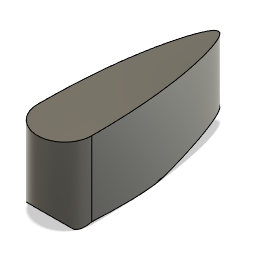
DLG_Höhenruder_träger (Autodesk Fusion 360 design; units mm, degrees)
Autodesk Fusion 360 part; units mm, degrees
sketch "Skizze1" plane through (0, 0, 0) normal (0, 0, 1) x (1, 0, 0)
  line L0 (6, 10) -> (-6, 10)
  line L1 (-6, 10) -> (-6, -10)
  line L2 (-6, -10) -> (6, -10)
  line L3 (6, -10) -> (6, 10)
  line L4 (6, 10) -> (-6, -10) construction
  line L5 (-6, 10) -> (6, -10) construction
  dimension "d1" = 12
  dimension "d2" = 20
  constraint horizontal L0
  constraint perpendicular L0 L1
  constraint parallel L0 L2
  constraint parallel L1 L3
  constraint coincident L4 origin
  constraint coincident L5 origin
  measures "d1" distance of L1.end L2.end
  measures "d2" distance of L0.end L1.end
extrude "Extrusion1" add sketch "Skizze1" along normal mid plane 40
sketch "Skizze2" plane through (0, 0, 20) normal (0, 0, 1) x (1, 0, 0)
  line L0 (6, -10) -> (6, 10)
  line L1 (6, 10) -> (-6, 10)
  line L2 (-6, 10) -> (-6, -10)
  line L3 (-6, -10) -> (6, -10)
  circle A0 centre (0, -10) radius 6.05
  dimension "d5" = 12.1
  constraint coincident L3 A0.centre
  constraint vertical origin A0.centre
  measures "d5" diameter of A0
sketch "Skizze3" plane through (0, 0, -20) normal (0, 0, -1) x (-1, 0, 0)
  line L0 (-6, 10) -> (-6, -10)
  line L1 (-6, -10) -> (6, -10)
  line L2 (6, -10) -> (6, 10)
  line L3 (6, 10) -> (-6, 10)
  circle A0 centre (0, -10) radius 6
  dimension "d6" = 12
  constraint coincident L0.end A0
  constraint coincident L1.end A0
  measures "d6" diameter of A0
loft "Erhebung1" cut profiles "Skizze2", "Skizze3" section 1 contours L0 L2 L3 A0 | L0 L2 L3 A0 section 2 contours L1 A0 | L1 A0
fillet "Abrundung1" radius 0.5 2 edges at (6, -9.6127, -10.0104) (-6, -9.6127, -10.0104)
sketch "Skizze4" plane through (0, 10, 0) normal (0, 1, 0) x (-1, 0, 0)
  line L0 (6, -20) -> (6, 20)
  line L1 (6, 20) -> (-6, 20)
  line L2 (-6, 20) -> (-6, -20)
  line L3 (-6, -20) -> (6, -20)
  spline S0 degree 5 poles (6, 14) (6, 11.3947) (5.9097, 6.4186) (5.5039, -0.3419) (4.5002, -7.9333) (2.887, -14.931) (1.2939, -19.2597) (0, -20.7369) (-1.2939, -19.2597) (-2.887, -14.931) (-4.5002, -7.9333) (-5.5039, -0.3419) (-5.9097, 6.4186) (-6, 11.3947) (-6, 14) knots 0 0 0 0 0 0 0.1 0.2 0.3 0.4 0.5 0.6 0.7 0.8 0.9 1 1 1 1 1 1
  arc A0 (6, 14) -> (-6, 14) centre (0, 14) ccw
  line L4 (0.5, -20) -> (-0.5, -20)
  line L5 (-6, 7.0737) -> (-6, 20.9263)
  line L6 (6, 20.9263) -> (6, 7.0737)
  point P0 (0, -20)
  dimension "d9" = 1
  constraint tangent L0 A0
  constraint vertical origin A0.centre
  constraint tangent L1 A0
  constraint midpoint L3 P0
  constraint tangent S0 A0
  constraint midpoint P0 L4
  constraint collinear L3 L4
  constraint midpoint S0.end L5
  constraint collinear L2 L5
  constraint midpoint S0.start L6
  constraint equal L5 L6
  measures "d9" distance of L4.start L4.end
extrude "Extrusion2" cut sketch "Skizze4" against normal blind 18 contours L0 L3 S0 L4 L6 | L0 L1 A0 L6 | L2 L3 S0 L4 L5 | L1 L2 A0 L5
